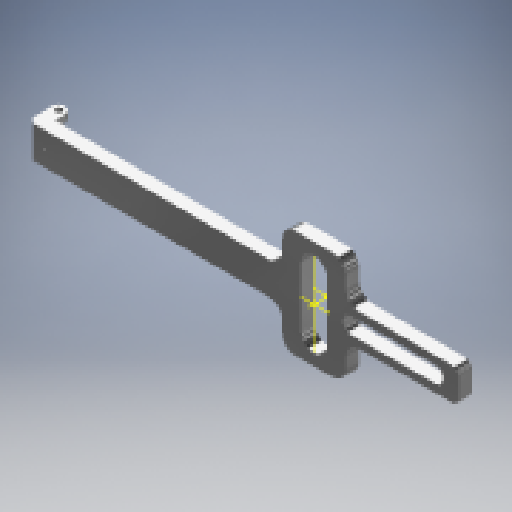
# Autodesk Inventor part: Scottish Yoke
Saved by Autodesk Inventor 2024.1 (Build 281209000, 209)
## iProperties
Created: 2008-06-06
Part Number: Scottish Yoke
Document SubType Name: Modeling
Designer: tangg
Density: 7.84 g/cm^3
Mass: 21.4252 g
Surface Area: 112.705 cm^2
Volume: 21.4252 cm^3
Stock Number: Scottish Yoke
Material: Steel, High Strength Low Alloy
Appearance: Chrome - Polished
Author: tangg
Autodesk Inventor part; units mm, degrees
ref_plane "YZ Plane" through (0, 0, 0) normal (1, 0, 0) x (0, 1, 0)
ref_plane "XY Plane" through (0, 0, 0) normal (0, 0, 1) x (1, 0, 0)
sketch "Sketch1" plane through (0, 0, 0) normal (0, 0, 1) x (1, 0, 0)
  line L0 (195.2625, 4.445) -> (195.2625, -4.445)
  line L1 (-7.9375, -7.62) -> (-7.9375, 7.62)
  circle A0 centre (0, 0) radius 0.4079
  arc A1 (195.2625, 4.445) -> (192.0875, 7.62) centre (192.0875, 4.445) ccw
  arc A2 (192.0875, -7.62) -> (195.2625, -4.445) centre (192.0875, -4.445) ccw
  line L2 (111.9187, 25.4) -> (142.0813, 25.4)
  line L3 (142.0813, -25.4) -> (111.9187, -25.4)
  line L4 (127, 42.8625) -> (127, -39.6875) construction
  line L5 (127, 19.8437) -> (127, 19.8437)
  line L6 (133.35, 13.4937) -> (133.35, -13.4937)
  line L7 (127, -19.8437) -> (127, -19.8437)
  line L8 (120.65, -13.4937) -> (120.65, 13.4938)
  arc A3 (127, 19.8437) -> (120.65, 13.4938) centre (127, 13.4937) ccw
  arc A4 (133.35, 13.4937) -> (127, 19.8437) centre (127, 13.4937) ccw
  arc A5 (127, -19.8437) -> (133.35, -13.4937) centre (127, -13.4937) ccw
  arc A6 (120.65, -13.4937) -> (127, -19.8437) centre (127, -13.4937) ccw
  line L9 (-7.9375, 7.62) -> (111.9187, 7.62)
  line L10 (142.0813, 7.62) -> (192.0875, 7.62)
  line L11 (192.0875, -7.62) -> (142.0813, -7.62)
  line L12 (111.9187, -7.62) -> (-7.9375, -7.62)
  line L13 (111.9187, -25.4) -> (111.9187, -7.62)
  line L14 (111.9187, 7.62) -> (111.9187, 25.4)
  line L15 (142.0813, 25.4) -> (142.0813, 7.62)
  line L16 (142.0813, -7.62) -> (142.0813, -25.4)
  point P0 (-7.9375, 0)
  point P1 (127, 25.4)
  point P2 (111.9187, 0)
  point P3 (120.65, 0)
  dimension "d0" = 15.24
  dimension "d1" = 203.2
  dimension "d2" = 3.175
  dimension "d3" = 127
  dimension "d4" = 6.35
  dimension "d43" = 25.4
  dimension "d44" = 25.4
  constraints: 34 end point, 14 tangent, 12 point on circle, 7 centre point, 4 equal radius, 4 midpoint, 3 horizontal alignment, 2 point on line, 1 coincident
  measures "d0" distance of L1.start L1.end
  measures "d1" distance between parallel lines of L0 L1
  measures "d2" radius of A1
  measures "d3" distance from line of L4 point (0, 0)
  measures "d4" radius of A3
  measures "d43" distance from line of point (120.65, 0) L2
  measures "d44" distance of point (111.919, 0) L3.end
extrude "Extrusion1" add sketch "Sketch1" along normal blind 6.35
ref_plane "Work Plane3" through (127, 7.62, 0) normal (1, 0, 0) x (0, 0, -1)
fillet "Fillet1" radius 6.35 8 edges at (142.0813, -25.4, 3.175) (111.9187, -25.4, 3.175) (142.0813, 25.4, 3.175) (111.9187, 25.4, 3.175) (142.0813, -7.62, 3.175) (111.9187, -7.62, 3.175) (111.9187, 7.62, 3.175) (142.0813, 7.62, 3.175)
sketch "Sketch10" plane through (0, 0, 6.35) normal (0, 0, 1) x (1, 0, 0)
  line L0 (144.0488, 3.81) -> (184.4165, 3.81)
  line L1 (187.5915, 0.635) -> (187.5915, -0.635)
  line L2 (184.4165, -3.81) -> (144.0488, -3.81)
  line L3 (140.8738, -0.635) -> (140.8738, 0.635)
  arc A0 (111.9187, -19.05) -> (118.2688, -25.4) centre (118.2688, -19.05) ccw projected
  line L4 (135.7313, -25.4) -> (118.2688, -25.4) projected
  arc A1 (135.7313, -25.4) -> (142.0813, -19.05) centre (135.7313, -19.05) ccw projected
  arc A2 (148.4313, -7.62) -> (142.0813, -13.97) centre (148.4313, -13.97) ccw projected
  line L5 (192.0875, -7.62) -> (148.4313, -7.62) projected
  arc A3 (192.0875, -7.62) -> (195.2625, -4.445) centre (192.0875, -4.445) ccw projected
  line L6 (195.2625, 4.445) -> (195.2625, -4.445) projected
  arc A4 (195.2625, 4.445) -> (192.0875, 7.62) centre (192.0875, 4.445) ccw projected
  line L7 (148.4313, 7.62) -> (192.0875, 7.62) projected
  arc A5 (142.0813, 13.97) -> (148.4313, 7.62) centre (148.4313, 13.97) ccw projected
  arc A6 (142.0813, 19.05) -> (135.7313, 25.4) centre (135.7313, 19.05) ccw projected
  line L8 (118.2687, 25.4) -> (135.7313, 25.4) projected
  arc A7 (118.2687, 25.4) -> (111.9187, 19.05) centre (118.2687, 19.05) ccw projected
  arc A8 (105.5687, 7.62) -> (111.9187, 13.97) centre (105.5687, 13.97) ccw projected
  line L9 (-7.9375, 7.62) -> (105.5687, 7.62) projected
  line L10 (-7.9375, -7.62) -> (-7.9375, 7.62) projected
  line L11 (105.5687, -7.62) -> (-7.9375, -7.62) projected
  arc A9 (111.9187, -13.97) -> (105.5687, -7.62) centre (105.5687, -13.97) ccw projected
  arc A10 (133.35, 13.4937) -> (120.65, 13.4938) centre (127, 13.4937) ccw projected
  line L12 (133.35, 13.4937) -> (133.35, -13.4937) projected
  arc A11 (120.65, -13.4937) -> (133.35, -13.4937) centre (127, -13.4937) ccw projected
  line L13 (120.65, -13.4937) -> (120.65, 13.4938) projected
  circle A12 centre (0, 0) radius 0.4079 projected
  line L14 (-7.9375, 7.62) -> (82.3369, 7.62)
  line L15 (82.3369, 7.62) -> (89.9679, 7.62)
  line L16 (195.2625, 4.445) -> (195.2625, -4.445) projected
  arc A13 (144.0488, 3.81) -> (140.8738, 0.635) centre (144.0488, 0.635) ccw
  arc A14 (140.8738, -0.635) -> (144.0488, -3.81) centre (144.0488, -0.635) ccw
  arc A15 (187.5915, 0.635) -> (184.4165, 3.81) centre (184.4165, 0.635) ccw
  arc A16 (184.4165, -3.81) -> (187.5915, -0.635) centre (184.4165, -0.635) ccw
  line L17 (-7.9375, 0) -> (195.2625, 0)
  line L18 (-7.9375, -7.62) -> (82.3369, -7.62)
  line L19 (82.3369, -7.62) -> (89.9679, -7.62)
  line L20 (142.0813, -13.97) -> (142.0813, -19.05) projected
  line L21 (142.0813, 19.05) -> (142.0813, 13.97) projected
  line L22 (111.9187, 13.97) -> (111.9187, 19.05) projected
  line L23 (111.9187, -19.05) -> (111.9187, -13.97) projected
  point P0 (187.5915, 0)
  point P1 (140.8738, 0)
  dimension "d22" = 3.175
  dimension "d23" = 7.62
  dimension "d24" = 3.175
  dimension "d25" = 7.62
  dimension "d26" = 7.62
  constraints: 18 end point, 8 point on circle, 8 tangent, 4 centre point, 4 midpoint, 4 point on line, 2 equal radius, 2 horizontal alignment, 1 horizontal, 1 parallel
  measures "d22" radius of A13
  measures "d23" distance between parallel lines of L2 L0
  measures "d24" radius of A15
  measures "d25" distance from line of point (0, 0) L14
  measures "d26" distance of L18.start L17.start
extrude "Extrusion7" cut sketch "Sketch10" against normal through all contours L0 A15 L1 L17 L3 A13 | L17 L1 A16 L2 A14 L3
sketch "Sketch7" plane through (0, 0, 0) normal (0, 1, 0) x (-1, 0, 0)
  line L0 (7.9375, 0) -> (7.9375, -5)
  line L1 (7.9375, 0) -> (-19.05, 0)
  line L2 (-111.9187, 0) -> (7.9375, 0) projected
  line L3 (7.9375, 0) -> (1.5875, 0)
  line L4 (1.5875, 0) -> (1.5875, -5)
  line L5 (7.9375, -5) -> (7.9375, 0)
  arc A0 (1.5875, -5) -> (7.9375, -5) centre (4.7625, -5) ccw
  circle A1 centre (4.7625, -5) radius 1.5875
  line L6 (1.5875, -5) -> (3.175, -5)
  line L7 (6.35, -5) -> (7.9375, -5)
  line L8 (7.9375, 0) -> (-111.9187, 0) projected
  point P0 (0, 0)
  point P1 (-89.9679, 0)
  dimension "d35" = 6.35
  dimension "d40" = 5
  dimension "d41" = 3.175
  dimension "d42" = 3.175
  constraints: 14 end point, 4 point on circle, 2 centre point, 2 coincident, 2 collinear, 2 parallel, 1 point on line, 1 vertical
  measures "d35" distance of L2.end L3.end
  measures "d40" distance of L0.start L0.end
  measures "d41" radius of A0
  measures "d42" diameter of A1
extrude "Extrusion9" add sketch "Sketch7" along normal mid plane 15.24 contours L0 L7 A1 L6 L4 L1 | A0 L6 A1 L7
sketch "Sketch12" plane through (0, 0, 0) normal (0, 1, 0) x (-1, 0, 0)
  line L0 (1.5875, 0) -> (7.9375, 0)
  arc A0 (1.5875, -5) -> (7.9375, -5) centre (4.7625, -5) ccw projected
  arc A1 (1.5875, -5) -> (7.9375, -5) centre (4.7625, -5) ccw projected
  line L1 (7.9375, 6.35) -> (7.9375, -5) projected
  line L2 (1.5875, -5) -> (1.5875, 0) projected
  point P0 (0, 0)
  constraints: 2 end point, 1 point on line
extrude "Extrusion11" cut sketch "Sketch12" against normal mid plane 7.62
chamfer "Chamfer1" distance 2.54 angle 45 1 edges at (-7.9375, 0, 6.35)
body "Solid1"
